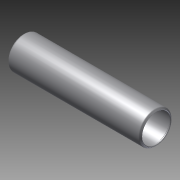
# Autodesk Inventor part: 04R-3.2570
Saved by Autodesk Inventor 2012 (Build 160160000, 160)
## iProperties
Created: 2013-01-17
Part Number: 04R-3.2570
Material: Default
Catalog Web Link: www.cadenas.de
Description: Tube-Original Line - Standard Air Cylinders
Vendor: BIMBA
Document SubType Name: Modeling
Designer: William
Manufacturer: BIMBA
Density: 1 g/cm^3
Category: PARTsolutions
Company: BIMBA
Title: 04R-3.2570
Author: Cadenas PARTsolutions
Comments: Original Line - Standard Air Cylinders
PSOL_IDENT_0: {\\10.0.0.242\data_v9\23d-libs\bimba\bimba\bimba_imperial\bimba_full_line\original_line_cylinders\st
PSOL_IDENT_1: andard_air_cylinders\tube.prj},188 {VTYP=3D},{NB=04R-3.2570},{LINA=04R-3.2570},{NN=Tube},{DATE=20.08
PSOL_IDENT_2: .2011 07:16:50},{GEOMDATE=18.02.2011 00:00:00},{VERSION=},{LINEID=40},{LINESUBID=-1},{WBVAR=MNT,ACTI
PSOL_IDENT_3: NG,NR,L,FOURHOLES,SR}  {NB=04R-3.2570},{LINA=04R-3.2570},{KT=DUMMY},{PN=04R-3.2570},{BORE=0.75000000
PSOL_IDENT_4: },{BOREPN=04},{MNT=},{MNTALG='' , 'Front Nose' , 'BF' , 'Front Block' , 'BFT' , 'Front Trunnion' , '
PSOL_IDENT_5: A' , 'Adjustable Stroke'},{ACTING=R},{ACTINGALG= '' , 'Single Acting' , 'R' , 'Reverse/Double Acting
PSOL_IDENT_6: ' },{NR=},{NRALG= '' , 'N/A' },{L=3.2570},{OD=0.8075},{ODN=0.8050},{ODP=0.8625},{ODB=0.8325},{ID=0.7
PSOL_IDENT_7: 615},{DV=0.00000000},{LV=0.00000000},{LV1=0.00000000},{G=0.0300},{FOURHOLES=0},{AA=0.3750},{BB=0.094
PSOL_IDENT_8: 0},{SR=},{SRALG= 'C' , 'Carbon Steel Rod' , 'SR' , '303 Stainless Steel Rod' , '' , '303 Stainless S
PSOL_IDENT_9: teel Rod'}
CNS_NT: Original Line - Standard Air Cylinders
CNS_NB: 04R-3.2570
CNS_NBSYN: $PN.
CNS_LINA: 04R-3.2570
CNS_PN: 04R-3.2570
CNS_BORE: 3/4
CNS_BOREPN: 04
CNS_MNT: Front Nose
CNS_MNTALG: '' , 'Front Nose' , 'BF' , 'Front Block' , 'BFT' , 'Front Trunnion' , 'A' , 'Adjustable Stroke'
CNS_ACTING: Reverse/Double Acting
CNS_ACTINGALG: '' , 'Single Acting' , 'R' , 'Reverse/Double Acting'
CNS_NR: N/A
CNS_NRALG: '' , 'N/A'
CNS_L: 3.2570
CNS_OD: 0.8075
CNS_ODN: 0.8050
CNS_ODP: 0.8625
CNS_ODB: 0.8325
CNS_ID: 0.7615
CNS_DV: 0.00000000
CNS_LV: 0.00000000
CNS_LV1: 0.00000000
CNS_G: 0.0300
CNS_FOURHOLES: 0
CNS_AA: 0.3750
CNS_BB: 0.0940
CNS_SR: 303 Stainless Steel Rod
CNS_SRALG: 'C' , 'Carbon Steel Rod' , 'SR' , '303 Stainless Steel Rod' , '' , '303 Stainless Steel Rod'
SUPPLIER: BIMBA
ARTICLENO: 04R-3.2570
BOMINFO: 04R-3.2570
CREATOR: CADENAS GmbH
Autodesk Inventor part; units mm, degrees
sketch "Sketch_1" plane through (0, 0, 0) normal (0, 0, 1) x (1, 0, 0)
  line L0 (82.7278, 0) -> (0, 0)
  arc A0 (-0.6395, 9.3472) -> (-0.6395, 9.1676) centre (-0.5497, 9.2574) ccw
  line L1 (-0.6395, 9.1676) -> (-0.381, 8.9091)
  line L2 (-0.381, 8.9091) -> (0, 8.9091)
  line L3 (0, 8.9091) -> (0.762, 9.671)
  line L4 (0.762, 9.671) -> (81.9658, 9.671)
  line L5 (81.9658, 9.671) -> (82.7278, 8.9091)
  line L6 (82.7278, 8.9091) -> (83.1088, 8.9091)
  line L7 (83.1088, 8.9091) -> (83.3673, 9.1676)
  arc A1 (83.3673, 9.1676) -> (83.3673, 9.3472) centre (83.2775, 9.2574) ccw
  line L8 (83.3673, 9.3472) -> (82.6824, 10.0321)
  arc A2 (82.6824, 10.0321) -> (82.1436, 10.2553) centre (82.1436, 9.4933) ccw
  line L9 (82.1436, 10.2553) -> (0.5842, 10.2553)
  arc A3 (0.5842, 10.2553) -> (0.0454, 10.0321) centre (0.5842, 9.4933) ccw
  line L10 (0.0454, 10.0321) -> (-0.6395, 9.3472)
  constraints: 22 end point, 8 point on circle, 4 centre point
revolve "Revolution1" add sketch "Sketch_1" angle 360 about axis through (82.7278, 0, 0) along (1, 0, 0)
ref_plane "tube_front_XY" through (0, 0, 0) normal (1, 0, 0) x (0, 0, -1)
ref_plane "tube_front_YZ" through (0, 0, 0) normal (0, 0, -1) x (0, 1, 0)
ref_plane "tube_front_ZX" through (0, 0, 0) normal (0, 1, 0) x (1, 0, 0)
ref_plane "tube_rear_XY" through (82.7278, 0, 0) normal (1, 0, 0) x (0, 0, -1)
ref_plane "tube_rear_YZ" through (82.7278, 0, 0) normal (0, 0, -1) x (0, 1, 0)
ref_plane "tube_rear_ZX" through (82.7278, 0, 0) normal (0, 1, 0) x (1, 0, 0)
ref_plane "cp1_XY" through (41.3639, 10.2553, 0) normal (1, 0, 0) x (0, 0, -1)
ref_plane "cp1_YZ" through (41.3639, 10.2553, 0) normal (0, 0, -1) x (0, 1, 0)
ref_plane "cp1_ZX" through (41.3639, 10.2553, 0) normal (0, 1, 0) x (1, 0, 0)
ref_plane "cp2_XY" through (41.3639, 0, -10.2553) normal (1, 0, 0) x (0, 0, -1)
ref_plane "cp2_YZ" through (41.3639, 0, -10.2553) normal (0, 0, -1) x (0, 1, 0)
ref_plane "cp2_ZX" through (41.3639, 0, -10.2553) normal (0, 1, 0) x (1, 0, 0)
ref_plane "cp3_XY" through (41.3639, -10.2553, 0) normal (1, 0, 0) x (0, 0, -1)
ref_plane "cp3_YZ" through (41.3639, -10.2553, 0) normal (0, 0, -1) x (0, 1, 0)
ref_plane "cp3_ZX" through (41.3639, -10.2553, 0) normal (0, 1, 0) x (1, 0, 0)
ref_plane "cp4_XY" through (41.3639, 0, 10.2553) normal (1, 0, 0) x (0, 0, -1)
ref_plane "cp4_YZ" through (41.3639, 0, 10.2553) normal (0, 0, -1) x (0, 1, 0)
ref_plane "cp4_ZX" through (41.3639, 0, 10.2553) normal (0, 1, 0) x (1, 0, 0)
body "Solid1"
